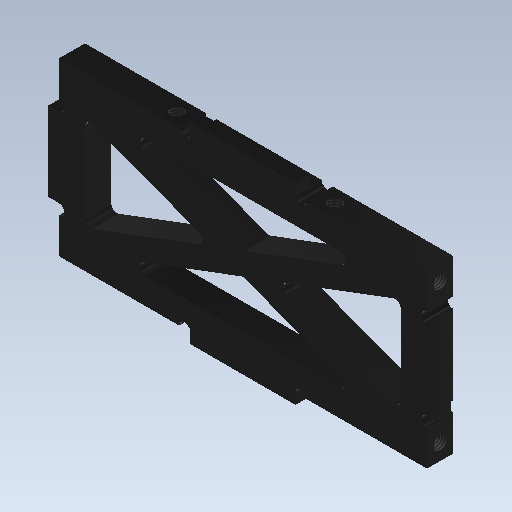
# Autodesk Inventor part: 胴体_メインフレーム_1_13
Saved by Autodesk Inventor 2020.4 (Build 244396000, 396)
## iProperties
Created: 2016-05-21
Part Number: 胴体_メインフレーム_1_13
Material: アセタール樹脂、黒
Document SubType Name: Modeling
Designer: hiroaki
Density: 1.425 g/cm^3
Appearance: 滑らか - 黒
Mass: 9.76521 g
Surface Area: 55.2384 cm^2
Volume: 6.85278 cm^3
Category: 胴体
d0: 1.050 mm
d1: 32.500 mm
d2: 70.000 mm
d3: 40.000 mm
d0_1: 15.000 mm
d1_1: 3.100 mm
d4: 5.000 mm
d7: 22.000 mm
d8: 16.000 mm
d9: 12.000 mm
d10: 51.500 mm
d11: 27.000 mm
d12: 1.000 mm
d13: 2.700 mm
d15: 92.000 mm
d16: 10.100 mm
d17: 36.500 mm
d18: 24.250 mm
d19: 2.400 mm
d20: 4.000 ul
d22: 360.00 deg
d24: 5.000 mm
d25: 3.100 mm
d26: 5.000 mm
d27: 5.000 mm
d28: 3.000 mm
d29: 8.000 mm
d32: 5.000 mm
d35: 4.000 mm
d36: 4.000 mm
d37: 4.000 mm
d38: 39.000 mm
d39: 30.000 mm
d41: 4.000 mm
d42: 5.000 mm
d43: 15.000 mm
d44: 3.100 mm
d47: 3.100 mm
d48: 26.500 mm
d50: 5.000 mm
d51: 2.100 mm
d52: 5.000 mm
d21: 32.500 mm
d23: 2.000 mm
d30: 2.000 mm
d34: 8.750 mm
d53: 20.000 mm
d54: 3.100 mm
d55: 5.000 mm
d56: 5.000 mm
d57: 0.00 deg
d58: 2.500 mm
d59: 0.00 deg
d60: 5.000 mm
d62: 2.500 mm
d66: 2.500 mm
d70: 2.500 mm
d74: 2.500 mm
Author: hiroaki
Autodesk Inventor part; units mm, degrees
ref_plane "YZ Plane" through (0, 0, 0) normal (1, 0, 0) x (0, 1, 0)
ref_plane "XZ Plane" through (0, 0, 0) normal (0, 1, 0) x (-1, 0, 0)
ref_plane "XY Plane" through (0, 0, 0) normal (0, 0, 1) x (1, 0, 0)
sketch "スケッチ1" plane through (0, 0, 0) normal (0, 0, 1) x (1, 0, 0)
  line L0 (-35, 9.6) -> (-35, 16.25)
  line L1 (-35, 16.25) -> (-20, 16.25)
  line L2 (20, 16.25) -> (35, 16.25)
  line L3 (35, 16.25) -> (35, 9.6)
  line L4 (0, 0) -> (0, 16.25) construction
  line L5 (0, 0) -> (37, 0) construction
  line L6 (35, 7.5) -> (37, 7.5)
  line L7 (37, 7.5) -> (37, -7.5)
  line L8 (37, -7.5) -> (35, -7.5)
  line L9 (-20, -16.25) -> (20, -16.25) construction
  line L10 (20, -16.25) -> (20, 16.25) construction
  line L11 (20, 16.25) -> (-20, 16.25) construction
  line L12 (-20, 16.25) -> (-20, -16.25) construction
  line L13 (-20, -16.25) -> (20, 16.25) construction
  line L14 (20, -16.25) -> (-20, 16.25) construction
  line L15 (-35, -16.25) -> (35, -16.25) construction
  line L16 (35, -16.25) -> (35, 16.25) construction
  line L17 (35, 16.25) -> (-35, 16.25) construction
  line L18 (-35, 16.25) -> (-35, -16.25) construction
  line L19 (-35, -16.25) -> (35, 16.25) construction
  line L20 (35, -16.25) -> (-35, 16.25) construction
  arc A0 (35, 9.6) -> (35, 7.5) centre (35, 8.55) ccw
  arc A1 (35, -7.5) -> (35, -9.6) centre (35, -8.55) ccw
  line L21 (35, -9.6) -> (35, -16.25)
  line L22 (35, -16.25) -> (20, -16.25)
  line L23 (20, -16.25) -> (12.1, -16.25)
  line L24 (-20, 16.25) -> (-12.1, 16.25)
  line L25 (-10, 16.25) -> (-10, 18.25)
  line L26 (-10, 18.25) -> (10, 18.25)
  line L27 (10, 18.25) -> (10, 16.25)
  line L28 (20, 16.25) -> (12.1, 16.25)
  arc A2 (-12.1, 16.25) -> (-10, 16.25) centre (-11.05, 16.25) ccw
  arc A3 (10, 16.25) -> (12.1, 16.25) centre (11.05, 16.25) ccw
  line L29 (-35, 7.5) -> (-37, 7.5)
  line L30 (-37, 7.5) -> (-37, -7.5)
  line L31 (-37, -7.5) -> (-35, -7.5)
  arc A4 (-35, 7.5) -> (-35, 9.6) centre (-35, 8.55) ccw
  arc A5 (-35, -9.6) -> (-35, -7.5) centre (-35, -8.55) ccw
  line L32 (-35, -9.6) -> (-35, -16.25)
  line L33 (-35, -16.25) -> (-20, -16.25)
  line L34 (-20, -16.25) -> (-12.1, -16.25)
  line L35 (-10, -16.25) -> (-10, -18.25)
  line L36 (-10, -18.25) -> (10, -18.25)
  line L37 (10, -18.25) -> (10, -16.25)
  arc A6 (-10, -16.25) -> (-12.1, -16.25) centre (-11.05, -16.25) ccw
  arc A7 (12.1, -16.25) -> (10, -16.25) centre (11.05, -16.25) ccw
  line L38 (-16.55, 19.1799) -> (-13.45, 19.1799) construction
  line L39 (-13.45, 19.1799) -> (-13.45, 12.4242) construction
  line L40 (-13.45, 12.4242) -> (-16.55, 12.4242) construction
  line L41 (-16.55, 12.4242) -> (-16.55, 19.1799) construction
  line L42 (-15, 19.1799) -> (-15, 12.4242) construction
  point P0 (0, 18.25)
  point P1 (0, 0)
  dimension "d0" = 1.05
  dimension "d1" = 32.5
  dimension "d2" = 70
  dimension "d3" = 40
  dimension "d23" = 2
  dimension "d30" = 2
  dimension "d34" = 8.75
  dimension "d53" = 20
  dimension "d54" = 3.1
  dimension "d55" = 5
  dimension "d85" = 32.5
  constraints: 86 end point, 17 point on line, 16 point on circle, 12 perpendicular, 9 midpoint, 8 centre point, 7 equal radius, 7 parallel, 6 horizontal, 6 symmetric about line, 5 tangent, 4 collinear, 2 vertical, 2 vertical alignment, 1 other
  measures "d0" radius of A0
  measures "d1" distance between parallel lines of L9 L11
  measures "d2" distance of L2.end L0.end
  measures "d3" distance between parallel lines of L10 L12
  measures "d23" distance of L6.start L6.end
  measures "d30" distance between parallel lines of L26 L11
  measures "d34" distance between parallel lines of L17 L29
  measures "d53" distance of L25.end L26.end
  measures "d54" distance of L38.start L38.end
  measures "d55" distance between parallel lines of L25 L42
  measures "d85" distance between parallel lines of L15 L17
extrude "押し出し1" add sketch "スケッチ1" along normal blind 5
sketch "スケッチ2" plane through (0, 0, 0) normal (0, 0, -1) x (-1, 0, 0)
  line L0 (35, 9.6) -> (35, 16.25) projected
  line L1 (-35, 16.25) -> (-35, 9.6) projected
  line L2 (-43.1427, 17.3125) -> (-35, 17.3125)
  line L3 (-35, 17.3125) -> (-35, -16.751)
  line L4 (-35, -16.751) -> (-43.1427, -16.751)
  line L5 (-43.1427, -16.751) -> (-43.1427, 17.3125)
  line L6 (35, 21.1805) -> (40.858, 21.1805)
  line L7 (40.858, 21.1805) -> (40.858, -13.6193)
  line L8 (40.858, -13.6193) -> (35, -13.6193)
  line L9 (35, -13.6193) -> (35, 21.1805)
  line L10 (-20, -16.25) -> (-12.1, -16.25)
  line L11 (-17.1371, 25.1848) -> (11.8342, 25.1848)
  line L12 (11.8342, 25.1848) -> (11.8342, 16.25)
  line L13 (11.8342, 16.25) -> (-17.1371, 16.25)
  line L14 (-17.1371, 16.25) -> (-17.1371, 25.1848)
  line L15 (-13.151, -21.5857) -> (17.7795, -21.5857)
  line L16 (17.7795, -21.5857) -> (17.7795, -16.25)
  line L17 (17.7795, -16.25) -> (-13.151, -16.25)
  line L18 (-13.151, -16.25) -> (-13.151, -21.5857)
  line L19 (-12.1, 16.25) -> (-35, 16.25)
  line L20 (-35, -16.25) -> (-12.1, -16.25)
  point P0 (0, 0)
  constraints: 38 end point, 8 parallel, 4 horizontal, 4 perpendicular, 3 collinear
extrude "押し出し2" cut sketch "スケッチ2" against normal blind 2.5
sketch "スケッチ3" plane through (12.1, 16.25, 0) normal (0, 1, 0) x (1, 0, 0)
  line L0 (-2.1, 0) -> (-2.1, -5) projected
  line L1 (-2.1, -5) -> (-22.1, -5) construction
  line L2 (-12.1, -5) -> (-12.1, 7.4607) construction
  line L3 (22.9, 0) -> (22.9, -5) projected
  point P0 (-12.1, 0)
  point P1 (2.9, -2.5)
  point P2 (-27.1, -2.5)
  point P3 (22.9, -2.5)
  dimension "d60" = 5
  constraints: 2 end point, 2 horizontal alignment, 2 midpoint, 1 symmetric about line, 1 vertical
  measures "d60" distance from line of L0 point (2.9, -2.5)
hole "穴1" at (15, 16.25, 2.5) at (-15, 16.25, 2.5) direction (0, -1, 0) diameter 2.459 depth 2.5 thread size "M3x0.5" class "6H" standard "ISO Metric profile"
mirror "ミラー1" about plane through (0, 0, 0) normal (0, 1, 0) of "穴1"
sketch "スケッチ4" plane through (35, -16.25, 5) normal (1, 0, 0) x (0, 0, -1)
  line L0 (5, 16.25) -> (0, 16.25) construction
  line L1 (0, 23.75) -> (0, 8.75) construction
  line L2 (5, 6.65) -> (0, 6.65) projected
  line L3 (5, 0) -> (0, 0) projected
  point P0 (2.5, 3)
  point P1 (2.5, 29.5)
  point P2 (2.5, 6.65)
  dimension "d86" = 3
  dimension "d87" = 26.5
  constraints: 2 end point, 2 midpoint, 2 vertical alignment, 1 symmetric about line
  measures "d86" distance from line of L3 point (2.5, 3)
  measures "d87" distance of point (2.5, 29.5) point (2.5, 3)
hole "穴2" at (35, -13.25, 2.5) at (35, 13.25, 2.5) direction (-1, 0, 0) diameter 2.459 depth 2.5 thread size "M3x0.5" class "6H" standard "ISO Metric profile"
mirror "ミラー2" about plane through (0, 0, 0) normal (1, 0, 0) of "穴2"
sketch "スケッチ5" plane through (0, 0, 0) normal (0, 0, -1) x (-1, 0, 0)
  line L0 (10, 16.25) -> (-10, 16.25) projected
  line L1 (-35, 7.5) -> (-35, 9.6) projected
  line L2 (-30, -11.25) -> (30, -11.25) construction
  line L3 (30, -11.25) -> (30, 11.25) construction
  line L4 (30, 11.25) -> (-30, 11.25) construction
  line L5 (-30, 11.25) -> (-30, -11.25) construction
  line L6 (-30, -11.25) -> (30, 11.25) construction
  line L7 (30, -11.25) -> (-30, 11.25) construction
  line L8 (-30, 9.114) -> (-30, -9.114)
  line L9 (-30, -9.114) -> (-5.696, 0)
  line L10 (-5.696, 0) -> (-30, 9.114)
  line L11 (-24.304, 11.25) -> (24.304, 11.25)
  line L12 (24.304, 11.25) -> (0, 2.136)
  line L13 (0, 2.136) -> (-24.304, 11.25)
  line L14 (-24.304, -11.25) -> (24.304, -11.25)
  line L15 (24.304, -11.25) -> (0, -2.136)
  line L16 (0, -2.136) -> (-24.304, -11.25)
  line L17 (30, 9.114) -> (30, -9.114)
  line L18 (30, -9.114) -> (5.696, 0)
  line L19 (5.696, 0) -> (30, 9.114)
  point P0 (-12.1, 16.25)
  point P1 (-20, 16.25)
  point P2 (-35, 16.25)
  point P3 (0, 0)
  dimension "d76" = 5
  dimension "d77" = 5
  dimension "d78" = 4
  dimension "d79" = 4
  dimension "d80" = 4
  dimension "d81" = 4
  constraints: 36 end point, 10 parallel, 4 collinear, 3 horizontal, 2 midpoint, 2 vertical, 1 perpendicular, 4 other
  measures "d76" distance between parallel lines of L4 L0
  measures "d77" distance between parallel lines of L1 L5
  measures "d78" distance between parallel lines of L19 L12
  measures "d79" distance between parallel lines of L15 L18
  measures "d80" distance between parallel lines of L10 L13
  measures "d81" distance between parallel lines of L16 L9
extrude "押し出し3" cut sketch "スケッチ5" against normal blind 10
fillet "フィレット1" radius 1.05 12 edges at (30, 9.114, 2.5) (30, -9.114, 2.5) (24.304, 11.25, 2.5) (5.696, 0, 2.5) (0, -2.136, 2.5) (0, 2.136, 2.5) (-30, -9.114, 2.5) (24.304, -11.25, 2.5) (-30, 9.114, 2.5) (-24.304, 11.25, 2.5) (-24.304, -11.25, 2.5) (-5.696, 0, 2.5)
equation "\"d85\" = d1"
equation "\"d60\" = d55"
equation "\"d77\" = d76"
equation "\"d79\" = d78"
equation "\"d80\" = d79"
equation "\"d81\" = d78"
equation "\"d52\" = 5"
